dadheadphonesv2 (Autodesk Fusion 360 design; units mm, degrees)
Autodesk Fusion 360 part; units mm, degrees
sketch "Sketch1" plane through (0, 0, 0) normal (0, 1, 0) x (1, 0, 0)
  line L0 (0, 0) -> (15, 0)
  line L1 (15, 0) -> (15, -7)
  line L2 (15, -7) -> (-37, -7)
  line L3 (-37, -7) -> (-37, -21.455)
  line L4 (-37, -21.455) -> (-44, -21.455)
  line L5 (-44, -21.455) -> (-44, 0)
  line L6 (-44, 0) -> (-7, 0)
  line L7 (-7, 0) -> (-7, 52)
  line L8 (-7, 52) -> (45, 52)
  line L9 (31, 35.5) -> (31, 42.5)
  line L10 (31, 42.5) -> (38, 42.5)
  line L11 (38, 42.5) -> (38, 45)
  line L12 (38, 45) -> (0, 45)
  line L13 (0, 45) -> (0, 0)
  line L14 (45, 35.5) -> (45, 52)
  line L15 (31, 35.5) -> (45, 35.5)
  line L16 (-7, 52) -> (-25.5, 0)
  line L17 (-7, 34.0996) -> (-19.1316, 0)
  dimension "d1" = 45
  dimension "d3" = 38
  dimension "d5" = 15
  dimension "d6" = 7
  dimension "d8" = 7
  dimension "d14" = 2.5
  dimension "d16" = 7
  dimension "d17" = 7
  dimension "d18" = 30
  dimension "d19" = 7
  dimension "d20" = 7
  dimension "d21" = 7
  dimension "d22" = 7
  dimension "d23" = 6
  constraint coincident L0.start L13.end
  constraint horizontal L0
  constraint perpendicular L0 L1
  constraint perpendicular L1 L2
  constraint perpendicular L2 L3
  constraint perpendicular L3 L4
  constraint perpendicular L4 L5
  constraint perpendicular L9 L10
  constraint perpendicular L10 L11
  constraint perpendicular L11 L12
  constraint perpendicular L0 L13
  constraint perpendicular L12 L13
  constraint perpendicular L9 L15
  constraint perpendicular L14 L15
  constraint perpendicular L8 L14
  constraint perpendicular L7 L8
  constraint perpendicular L6 L7
  constraint midpoint L6 L16.end
  constraint coincident L7 L17.start
  constraint coincident L6 L17.end
  constraint parallel L16 L17
  measures "d1" distance of L12.end L0.start
  measures "d3" distance of L11.end L12.end
  measures "d5" distance of L0.start L0.end
  measures "d6" distance of L9.end L10.end
  measures "d8" distance of L9.start L9.end
  measures "d14" vertical distance of L10.end L11.end
  measures "d16" distance of L11 L14
  measures "d17" distance of L8 L12
  measures "d18" distance of L3 L7
  measures "d19" distance of L7 L13
  measures "d20" distance of L2 L6
  measures "d21" distance of L0 L2
  measures "d22" distance of L3.end L4.end
  measures "d23" distance of L16 L17
extrude "Extrude1" add sketch "Sketch1" along normal blind 10 contours L0 L1 L2 L3 L4 L5 L6 L7 L8 L9 L10 L11 L12 L13 L14 L15 | L6 L7 L16 L17
